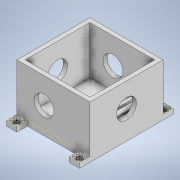
# Autodesk Inventor part: Wechsel_Hülle
Saved by Autodesk Inventor 2021 (Build 250183000, 183)
## iProperties
Created: 2021-01-25
Part Number: Wechsel_Hülle
Material: Generisch
Document SubType Name: Modeling
Designer: Jaro Machnow
Density: 1 g/cm^3
Appearance: Vorgabe
Author: Jaro Machnow
Autodesk Inventor part; units mm, degrees
ref_plane "YZ Plane" through (0, 0, 0) normal (1, 0, 0) x (0, 1, 0)
ref_plane "XZ Plane" through (0, 0, 0) normal (0, 1, 0) x (-1, 0, 0)
ref_plane "XY Plane" through (0, 0, 0) normal (0, 0, 1) x (1, 0, 0)
sketch "Skizze1" plane through (0, 0, 0) normal (0, 1, 0) x (-1, 0, 0)
  line L0 (35, 35) -> (-35, 35)
  line L1 (-35, 35) -> (-35, -35)
  line L2 (-35, -35) -> (35, -35)
  line L3 (35, -35) -> (35, 35)
  line L4 (0, 35) -> (0, -35) construction
  line L5 (35, 0) -> (-35, 0) construction
  point P0 (0, 0)
  point P1 (0, 0)
  dimension "d0" = 70
  dimension "d1" = 70
  constraints: 12 end point, 5 midpoint, 2 parallel, 1 coincident, 1 horizontal, 1 perpendicular
  measures "d0" distance of L2.end L1.end
  measures "d1" distance of L1.end L0.end
extrude "Extrusion1" add sketch "Skizze1" along normal blind 50
shell "Wandung1" thickness 4 removed faces 1 at (11.6667, 50, -11.6667)
sketch "Skizze2" plane through (35, 0, 35) normal (1, 0, 0) x (0, 0, -1)
  circle A0 centre (35, 27) radius 9.5
  line L0 (0, 0) -> (0, 50) construction
  line L1 (0, 0) -> (70, 0) construction
  line L2 (0, 50) -> (70, 0) construction
  line L3 (0, 50) -> (70, 50) construction
  line L4 (70, 50) -> (0, 0) construction
  point P0 (35, 0)
  point P1 (35, 25)
  point P2 (35, 25)
  dimension "d5" = 19
  dimension "d27" = 2
  constraints: 4 end point, 2 midpoint, 1 centre point, 1 vertical alignment
  measures "d5" diameter of A0
  measures "d27" distance of A0.centre point (35, 25)
sketch "Skizze3" plane through (35, 0, -35) normal (0, 0, -1) x (-1, 0, 0)
  circle A0 centre (44, 25) radius 9.5
  line L0 (0, 0) -> (0, 50) construction
  line L1 (70, 0) -> (70, 50) construction
  line L2 (0, 50) -> (70, 0) construction
  line L3 (0, 50) -> (70, 50) construction
  line L4 (0, 0) -> (70, 50) construction
  point P0 (35, 0)
  point P1 (35, 25)
  point P2 (35, 25)
  dimension "d6" = 19
  dimension "d11" = 9
  constraints: 4 end point, 2 midpoint, 1 centre point, 1 horizontal alignment
  measures "d6" diameter of A0
  measures "d11" distance of A0.centre point (35, 25)
extrude "Extrusion2" cut sketch "Skizze3" against normal blind 95.5
extrude "Extrusion3" cut sketch "Skizze2" against normal blind 10
sketch "Skizze4" plane through (-31, 4, -31) normal (0, 1, 0) x (1, 0, 0)
  line L0 (62, -62) -> (0, -62) projected
  line L1 (62, 0) -> (0, 0) projected
  line L2 (62, -62) -> (46, -62)
  line L3 (46, -62) -> (46, 0)
  line L4 (46, 0) -> (62, 0)
  line L5 (62, 0) -> (62, -62)
  point P0 (31, -31)
  dimension "d12" = 16
  constraints: 8 end point, 2 parallel, 1 horizontal, 1 perpendicular, 1 point on line
  measures "d12" distance of L3.end L4.end
extrude "Extrusion4" add sketch "Skizze4" along normal blind 11
sketch "Skizze5" plane through (-31, 15, -31) normal (0, 1, 0) x (1, 0, 0)
  line L0 (62, -62) -> (46, -62) projected
  line L1 (0, 0) -> (62, 0) projected
  line L2 (58, -62) -> (56, -62)
  line L3 (56, -62) -> (56, 0)
  line L4 (56, 0) -> (58, 0)
  line L5 (58, 0) -> (58, -62)
  line L6 (51, -62) -> (49, -62)
  line L7 (49, -62) -> (49, 0)
  line L8 (49, 0) -> (51, 0)
  line L9 (51, 0) -> (51, -62)
  line L10 (62, 0) -> (62, -62) projected
  line L11 (46, 0) -> (46, -62) projected
  line L12 (53.5, -62) -> (53.5, 0) construction
  point P0 (31, -31)
  point P1 (51, 0)
  point P2 (49, 0)
  point P3 (58, 0)
  dimension "d15" = 2
  dimension "d19" = 7.5
  dimension "d20" = 5
  constraints: 18 end point, 6 point on line, 4 parallel, 3 perpendicular, 2 horizontal, 2 other
  measures "d15" distance of L3.end L4.end
  measures "d19" distance between parallel lines of L11 L12
  measures "d20" distance between parallel lines of L3 L9
extrude "Extrusion5" cut sketch "Skizze5" against normal blind 3 contours L0 L3 L1 L5 | L0 L7 L1 L9
fillet "Rundung1" radius 1 4 edges at (27, 12, 0) (25, 12, 0) (20, 12, 0) (18, 12, 0)
sketch "Skizze6" plane through (-35, 0, -35) normal (-1, 0, 0) x (0, 0, 1)
  line L0 (70, 0) -> (70, 50) construction
  line L1 (70, 50) -> (0, 0) construction
  line L2 (0, 0) -> (70, 0) construction
  line L3 (70, 0) -> (0, 50) construction
  circle A0 centre (35, 25) radius 9.5
  point P0 (35, 0)
  dimension "d24" = 19
  constraints: 4 end point, 1 centre point, 1 midpoint
  measures "d24" diameter of A0
extrude "Extrusion6" cut sketch "Skizze6" against normal blind 10
sketch "Skizze7" plane through (-35, 0, 35) normal (0, 0, 1) x (1, 0, 0)
  line L0 (0, 0) -> (10, 0)
  line L1 (10, 0) -> (10, 5)
  line L2 (10, 5) -> (0, 5)
  line L3 (0, 5) -> (0, 0)
  point P0 (35, 0)
  dimension "d28" = 10
  dimension "d29" = 5
  constraints: 8 end point, 2 parallel, 1 horizontal, 1 perpendicular
  measures "d28" distance of L2.end L1.end
  measures "d29" distance of L1.end L0.end
extrude "Extrusion7" add sketch "Skizze7" along normal blind 10
sketch "Skizze8" plane through (-35, 5, 35) normal (0, 1, 0) x (1, 0, 0)
  line L0 (0, 0) -> (70, 0) construction
  line L1 (10, 0) -> (10, -10) construction
  line L2 (0, -10) -> (10, -10) construction
  line L3 (0, -10) -> (10, 0) construction
  line L4 (0, 70) -> (0, 0) construction
  line L5 (0, 0) -> (10, -10) construction
  point P0 (35, 35)
  point P1 (5, -5)
  constraints: 4 end point, 1 midpoint, 1 perpendicular
sketch "Skizze9" plane through (-35, 5, 35) normal (0, 1, 0) x (1, 0, 0)
  point P0 (5, -5)
sketch "Skizze10" plane through (-35, 50, 35) normal (0, 0, 1) x (1, 0, 0)
  line L0 (10, -50) -> (70, -50) projected
  line L1 (70, -50) -> (60, -50)
  line L2 (60, -50) -> (60, -45)
  line L3 (60, -45) -> (70, -45)
  line L4 (70, -45) -> (70, -50)
  point P0 (35, -50)
  dimension "d39" = 10
  dimension "d40" = 5
  constraints: 8 end point, 2 parallel, 1 horizontal, 1 perpendicular
  measures "d39" distance of L2.end L3.end
  measures "d40" distance of L1.end L2.end
extrude "Extrusion8" add sketch "Skizze10" along normal blind 10
sketch "Skizze11" plane through (35, 0, -35) normal (0, 0, -1) x (-1, 0, 0)
  line L0 (0, 0) -> (0, 50) projected
  line L1 (0, 0) -> (10, 0)
  line L2 (10, 0) -> (10, 5)
  line L3 (10, 5) -> (0, 5)
  line L4 (0, 5) -> (0, 0)
  line L5 (0, 0) -> (70, 0) projected
  line L6 (70, 0) -> (60, 0)
  line L7 (60, 0) -> (60, 5)
  line L8 (60, 5) -> (70, 5)
  line L9 (70, 5) -> (70, 0)
  point P0 (35, 0)
  dimension "d43" = 10
  dimension "d44" = 5
  dimension "d45" = 10
  dimension "d46" = 5
  constraints: 16 end point, 4 parallel, 2 horizontal, 2 perpendicular
  measures "d43" distance of L3.end L2.end
  measures "d44" distance of L2.end L1.end
  measures "d45" distance of L7.end L8.end
  measures "d46" distance of L6.end L7.end
extrude "Extrusion9" add sketch "Skizze11" along normal blind 10
sketch "Skizze12" plane through (25, 5, 35) normal (0, 1, 0) x (1, 0, 0)
  line L0 (0, 0) -> (0, -10) construction
  line L1 (-60, 0) -> (10, 0) construction
  line L2 (0, -10) -> (10, 0) construction
  line L3 (0, -10) -> (10, -10) construction
  line L4 (10, -10) -> (0, 0) construction
  line L5 (-60, -10) -> (-60, 80) construction
  line L6 (-50, 80) -> (-60, 80) construction
  line L7 (-60, 70) -> (-50, 80) construction
  line L8 (-60, 80) -> (-50, 70) construction
  line L9 (0, 70) -> (0, 80) construction
  line L10 (10, 80) -> (0, 80) construction
  line L11 (0, 70) -> (10, 80) construction
  line L12 (10, 70) -> (10, 80) construction
  line L13 (0, 80) -> (10, 70) construction
  point P0 (-25, 35)
  point P1 (5, -5)
  point P2 (5, 75)
  point P3 (-55, 75)
  constraints: 12 end point, 3 midpoint, 3 perpendicular, 1 point on line
sketch "Skizze13" plane through (25, 5, -35) normal (0, 1, 0) x (1, 0, 0)
  point P0 (5, 5)
  point P1 (5, -75)
  point P2 (-55, 5)
hole "Bohrung2" at (30, 5, -40) at (30, 5, 40) at (-30, 5, -40) direction (0, -1, 0) diameter 5.5 end through all countersink diameter 10.4 countersink angle 90
sketch "Skizze14" plane through (-35, 5, 35) normal (0, 1, 0) x (1, 0, 0)
  point P0 (5, -5)
hole "Bohrung3" at (-30, 5, 40) direction (0, -1, 0) diameter 5.5 end through all countersink diameter 10.4 countersink angle 90
